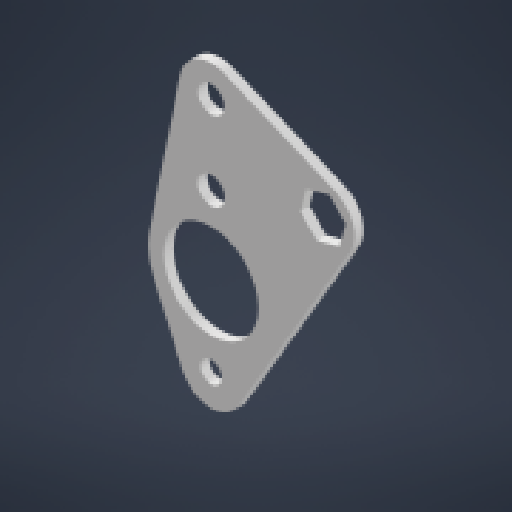
# Autodesk Inventor part: inner-pto-mount
Saved by Autodesk Inventor 2023.2 (Build 272271000, 271)
## iProperties
Created: 2023-03-24
Part Number: inner-pto-mount
Material: Generic
Document SubType Name: Modeling
Designer: Liam
Density: 1 g/cm^3
Appearance: Default
Author: Liam
Autodesk Inventor part; units mm, degrees
ref_plane "YZ Plane" through (0, 0, 0) normal (1, 0, 0) x (0, 1, 0)
ref_plane "XZ Plane" through (0, 0, 0) normal (0, 1, 0) x (-1, 0, 0)
ref_plane "XY Plane" through (0, 0, 0) normal (0, 0, 1) x (1, 0, 0)
sketch "Sketch1" plane through (0, 0, 0) normal (0, 0, 1) x (1, 0, 0)
  line L0 (20.7324, 65.9602) -> (21.7374, 69.6353) projected
  line L1 (17.0472, 64.993) -> (20.7324, 65.9602) projected
  line L2 (14.367, 67.7009) -> (17.0472, 64.993) projected
  line L3 (15.372, 71.376) -> (14.367, 67.7009) projected
  line L4 (19.0572, 72.3432) -> (15.372, 71.376) projected
  line L5 (21.7374, 69.6353) -> (19.0572, 72.3432) projected
  circle A0 centre (0, 63.5) radius 2.1844 projected
  circle A1 centre (0, 50.8) radius 7.62
  circle A2 centre (0, 38.1) radius 1.7272 projected
  line L6 (22.4264, 66.0849) -> (4.3742, 35.5168)
  line L7 (-4.6559, 36.068) -> (-9.3118, 46.736)
  line L8 (-4.6559, 36.068) -> (-9.3118, 46.736)
  line L9 (16.654, 73.5519) -> (-1.3982, 68.3838)
  line L10 (-9.3118, 54.864) -> (-4.6559, 65.532)
  line L11 (-9.3118, 46.736) -> (-4.6559, 36.068)
  arc A3 (-4.6559, 36.068) -> (4.3742, 35.5168) centre (0, 38.1) ccw
  arc A4 (-9.3118, 54.864) -> (-9.3118, 46.736) centre (0, 50.8) ccw
  arc A5 (-1.3982, 68.3838) -> (-4.6559, 65.532) centre (0, 63.5) ccw
  arc A6 (22.4264, 66.0849) -> (16.654, 73.5519) centre (18.0522, 68.6681) ccw
  point P0 (0, 0)
  dimension "d4" = 15.24
  constraints: 12 end point, 8 point on circle, 5 centre point, 4 tangent, 2 collinear
  measures "d4" diameter of A1
extrude "Extrusion1" add sketch "Sketch1" along normal blind 1.524
body "Solid1"
